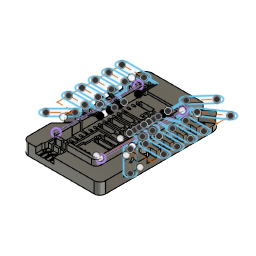
2020_10_06_Nano To Capacitive Sensors One Face Plus v2 (Autodesk Fusion 360 design; units mm, degrees)
Autodesk Fusion 360 part; units mm, degrees
note: some values were not read from the file. Chosen so that the rebuilt part matches the saved one: which face or edge a step refers to. Set by a fixed rule: which sketch regions a step uses.
(part 1 of 3)
sketch "ArduinoNano" plane through (0, 0, 0) normal (0, 0, 1) x (1, 0, 0)
  arc A0 (-13.9477, 42.08) -> (-13.9477, 42.68) centre (-14.2477, 42.38) ccw
  line L0 (-12.5236, 31.2001) -> (-12.133, 30.8096)
  line L1 (-6.271, 43.18) -> (-6.271, 42.88)
  line L2 (-4.5943, 36.68) -> (-4.7943, 36.48)
  line L3 (-13.9477, 42.68) -> (-13.7477, 42.88)
  line L4 (0, 0) -> (0, 43.18)
  line L5 (-6.771, 0) -> (0, 0)
  line L6 (-6.271, 41.88) -> (-6.271, 37.48)
  line L7 (-12.271, 36.18) -> (-12.271, 36.48)
  line L8 (-12.271, 37.48) -> (-12.271, 41.88)
  circle A1 centre (-7.271, 3.0017) radius 0.76
  circle A2 centre (-9.271, 3) radius 0.76
  circle A3 centre (-1.524, 19.156) radius 0.5
  arc A4 (-13.9477, 36.68) -> (-13.9477, 37.28) centre (-14.2477, 36.98) ccw
  line L9 (-6.3515, 30.7521) -> (-5.9609, 31.1427)
  line L10 (-1.524, 24.156) -> (-1.024, 24.156)
  line L11 (-6.271, 36.18) -> (-12.271, 36.18)
  line L12 (-12.271, 36.48) -> (-13.7477, 36.48)
  arc A5 (-13.7477, 37.48) -> (-12.271, 37.48) centre (-13.0093, 38.2183) ccw
  circle A6 centre (-1.524, 11.656) radius 0.5
  arc A7 (-4.7943, 41.88) -> (-6.271, 41.88) centre (-5.5326, 41.1416) ccw
  line L13 (-6.271, 42.88) -> (-4.7943, 42.88)
  line L14 (0, 43.18) -> (-6.271, 43.18)
  circle A8 centre (-1.524, 24.156) radius 0.889
  circle A9 centre (-1.524, 14.156) radius 0.889
  line L15 (-18.542, 43.18) -> (-18.542, 0)
  line L16 (-11.6107, 25.028) -> (-12.0012, 24.6374)
  arc A10 (-13.7477, 42.88) -> (-12.271, 42.88) centre (-13.0093, 43.6183) ccw
  circle A11 centre (-1.524, 9.156) radius 0.5
  circle A12 centre (-17.018, 11.656) radius 0.889
  line L17 (-12.271, 43.18) -> (-18.542, 43.18)
  line L18 (-4.7943, 42.88) -> (-4.5943, 42.68)
  line L19 (-13.7477, 41.88) -> (-13.9477, 42.08)
  arc A13 (-4.7943, 36.48) -> (-6.271, 36.48) centre (-5.5326, 35.7416) ccw
  line L20 (-4.5943, 42.08) -> (-4.7943, 41.88)
  arc A14 (-4.5943, 42.68) -> (-4.5943, 42.08) centre (-4.2943, 42.38) ccw
  line L21 (-6.271, 37.48) -> (-4.7943, 37.48)
  line L22 (-18.542, 0) -> (-11.771, 0)
  arc A15 (-4.5943, 37.28) -> (-4.5943, 36.68) centre (-4.2943, 36.98) ccw
  line L23 (-6.271, 36.48) -> (-6.271, 36.18)
  line L24 (-11.771, 0) -> (-6.771, 0)
  line L25 (-13.7477, 36.48) -> (-13.9477, 36.68)
  line L26 (-13.9477, 37.28) -> (-13.7477, 37.48)
  line L27 (-12.271, 41.88) -> (-13.7477, 41.88)
  line L28 (-4.7943, 37.48) -> (-4.5943, 37.28)
  line L29 (-6.0786, 0) -> (-12.4635, 0)
  circle A16 centre (-7.271, 0.9961) radius 0.76
  arc A17 (-6.8307, 32.2953) -> (-6.8307, 32.0124) centre (-6.9721, 32.1539) cw
  line L30 (-6.771, 13.9686) -> (-11.771, 13.9686)
  line L31 (0, 43.18) -> (-18.542, 43.18)
  line L32 (-12.133, 30.8096) -> (-12.4229, 30.5196)
  line L33 (-18.542, 43.18) -> (0, 43.18)
  circle A18 centre (-17.018, 6.656) radius 0.889
  line L34 (-12.271, 42.88) -> (-12.271, 43.18)
  line L35 (-12.7703, 26.1877) -> (-13.1609, 25.7971)
  line L36 (-6.771, 18.0694) -> (-6.771, 13.9686)
  line L37 (-15.829, 4.2) -> (-2.8014, 4.2)
  circle A19 centre (-1.524, 16.656) radius 0.5
  circle A20 centre (-17.018, 9.156) radius 0.889
  line L38 (-11.9006, 25.3179) -> (-11.6107, 25.028)
  arc A21 (-9.4003, 23.3921) -> (-9.5417, 23.4507) centre (-9.4003, 23.5921) cw
  circle A22 centre (-1.524, 39.156) radius 0.889
  line L39 (-8.0618, 33.5265) -> (-7.9903, 33.4549)
  circle A23 centre (-17.018, 16.656) radius 0.5
  line L40 (-12.4635, 4.2) -> (-6.0786, 4.2)
  circle A24 centre (-17.018, 6.656) radius 0.5
  arc A25 (-14.0589, 28.3093) -> (-14.0003, 28.4507) centre (-13.8589, 28.3093) cw
  line L41 (-5.6781, 31.1427) -> (-5.671, 31.1356)
  circle A26 centre (-17.018, 19.156) radius 0.5
  line L42 (-16.518, 19.156) -> (-17.018, 19.156)
  line L43 (-17.018, 12.156) -> (-17.018, 11.156)
  line L44 (-11.771, 13.9686) -> (-11.771, 18.0694)
  line L45 (-12.4229, 30.5196) -> (-12.8135, 30.9102)
  circle A27 centre (-17.018, 14.156) radius 0.889
  line L46 (-1.524, 19.156) -> (-1.024, 19.156)
  circle A28 centre (-1.524, 9.156) radius 0.889
  line L47 (-12.2912, 24.9274) -> (-11.9006, 25.3179)
  circle A29 centre (-17.018, 31.656) radius 0.889
  circle A30 centre (-1.524, 24.156) radius 0.5
  arc A31 (-12.8065, 31.2001) -> (-12.5236, 31.2001) centre (-12.665, 31.0587) cw
  line L48 (-1.524, 21.656) -> (-1.024, 21.656)
  line L49 (-12.2841, 24.6374) -> (-12.2912, 24.6445)
  arc A32 (-12.2912, 24.6445) -> (-12.2912, 24.9274) centre (-12.1497, 24.7859) cw
  line L50 (-11.771, 18.0694) -> (-6.771, 18.0694)
  circle A33 centre (-17.018, 4.156) radius 0.5
  circle A34 centre (-1.524, 6.656) radius 0.889
  arc A35 (-12.0012, 24.6374) -> (-12.2841, 24.6374) centre (-12.1427, 24.7789) cw
  line L51 (-7.271, 0.2361) -> (-7.271, 1.7561)
  line L52 (-5.671, 30.8528) -> (-6.0616, 30.4622)
  line L53 (-17.518, 11.656) -> (-16.518, 11.656)
  arc A36 (-5.9609, 31.1427) -> (-5.6781, 31.1427) centre (-5.8195, 31.0013) cw
  arc A37 (-12.8135, 30.9102) -> (-12.8135, 31.1931) centre (-12.6721, 31.0517) cw
  line L54 (-12.8135, 31.1931) -> (-12.8065, 31.2001)
  circle A38 centre (-17.018, 16.656) radius 0.889
  arc A39 (-5.671, 31.1356) -> (-5.671, 30.8528) centre (-5.8124, 30.9942) cw
  circle A40 centre (-17.018, 9.156) radius 0.5
  line L55 (-12.4635, 0) -> (-12.4635, 4.2)
  line L56 (-6.0616, 30.4622) -> (-6.3515, 30.7521)
  circle A41 centre (-17.018, 14.156) radius 0.5
  circle A42 centre (-1.524, 16.656) radius 0.889
  line L57 (-7.771, 0.9965) -> (-6.511, 0.9965)
  line L58 (-6.0786, 4.2) -> (-6.0786, 0)
  circle A43 centre (-1.524, 14.156) radius 0.5
  circle A44 centre (-17.018, 11.656) radius 0.5
  arc A45 (-4.5417, 28.4507) -> (-4.4831, 28.3093) centre (-4.6831, 28.3093) cw
  line L59 (-6.8881, 24.0072) -> (-6.8952, 24.0002)
  line L60 (-7.7579, 23.4203) -> (-8.1484, 23.8109)
  arc A46 (-9.0003, 23.4507) -> (-9.1417, 23.3921) centre (-9.1417, 23.5921) cw
  arc A47 (-9.1417, 32.9678) -> (-9.0003, 32.9093) centre (-9.1417, 32.7678) cw
  circle A48 centre (-11.2599, 1.0002) radius 0.76
  line L61 (-12.0199, 1.0002) -> (-10.4999, 1.0002)
  line L62 (-8.3809, 32.7815) -> (-8.7353, 33.1359)
  circle A49 centre (-1.524, 6.656) radius 0.5
  arc A50 (-5.7355, 25.1598) -> (-6.0184, 25.1598) centre (-5.8769, 25.3012) cw
  arc A51 (-7.9903, 33.4549) -> (-7.9903, 33.1721) centre (-8.1317, 33.3135) cw
  line L63 (-9.0003, 32.9093) -> (-4.5417, 28.4507)
  line L64 (-7.2212, 31.6218) -> (-7.5112, 31.9118)
  arc A52 (-6.5407, 31.7225) -> (-6.2579, 31.7225) centre (-6.3993, 31.5811) cw
  line L65 (-7.5112, 31.9118) -> (-7.1206, 32.3023)
  line L66 (-7.2787, 24.6807) -> (-6.8881, 24.2901)
  arc A53 (-13.1609, 25.7971) -> (-13.4437, 25.7971) centre (-13.3023, 25.9385) cw
  arc A54 (-3.9245, 29.3891) -> (-3.9245, 29.1063) centre (-4.0659, 29.2477) cw
  line L67 (-6.5982, 24.58) -> (-6.9888, 24.9706)
  line L68 (-13.4508, 26.087) -> (-13.0602, 26.4776)
  line L69 (-14.0003, 28.4507) -> (-9.5417, 32.9093)
  line L70 (-4.4831, 28.3093) -> (-4.4831, 28.0507)
  line L71 (-6.2579, 31.7225) -> (-6.2508, 31.7154)
  line L72 (-1.524, 34.156) -> (-1.024, 34.156)
  line L73 (-8.7353, 33.1359) -> (-8.3447, 33.5265)
  arc A55 (-7.4105, 32.8751) -> (-7.4105, 32.5923) centre (-7.5519, 32.7337) cw
  line L74 (-9.4003, 32.9678) -> (-9.1417, 32.9678)
  circle A56 centre (-1.524, 31.656) radius 0.5
  circle A57 centre (-1.524, 34.156) radius 0.5
  line L75 (-6.9313, 31.3319) -> (-6.5407, 31.7225)
  line L76 (-13.0602, 26.4776) -> (-12.7703, 26.1877)
  arc A58 (-8.3447, 33.5265) -> (-8.0618, 33.5265) centre (-8.2033, 33.385) cw
  line L77 (-5.4818, 29.8824) -> (-5.7717, 30.1723)
  arc A59 (-7.7004, 32.8822) -> (-7.4176, 32.8822) centre (-7.559, 32.7408) cw
  circle A60 centre (-1.524, 36.656) radius 0.5
  arc A61 (-14.0003, 27.9093) -> (-14.0589, 28.0507) centre (-13.8589, 28.0507) cw
  line L78 (-1.524, 39.156) -> (-1.024, 39.156)
  line L79 (-4.8587, 26.3195) -> (-5.2493, 26.7101)
  line L80 (-6.6414, 31.042) -> (-6.9313, 31.3319)
  arc A62 (-6.2508, 31.7154) -> (-6.2508, 31.4326) centre (-6.3922, 31.574) cw
  line L81 (-4.5417, 27.9093) -> (-9.0003, 23.4507)
  line L82 (-7.4176, 32.8822) -> (-7.4105, 32.8751)
  circle A63 centre (-11.269, 3) radius 0.76
  circle A64 centre (-1.524, 36.656) radius 0.889
  line L83 (-6.2508, 31.4326) -> (-6.6414, 31.042)
  line L84 (-13.4437, 25.7971) -> (-13.4508, 25.8042)
  line L85 (-6.8307, 32.0124) -> (-7.2212, 31.6218)
  arc A65 (-7.1206, 32.3023) -> (-6.8377, 32.3023) centre (-6.9791, 32.1609) cw
  line L86 (-17.518, 6.656) -> (-16.518, 6.656)
  circle A66 centre (-1.524, 4.156) radius 0.889
  line L87 (-7.9903, 33.1721) -> (-8.3809, 32.7815)
  line L88 (-9.1417, 23.3921) -> (-9.4003, 23.3921)
  circle A67 centre (-1.524, 4.156) radius 0.5
  line L89 (-7.4105, 32.5923) -> (-7.8011, 32.2017)
  line L90 (-1.524, 36.656) -> (-1.024, 36.656)
  arc A68 (-13.4508, 25.8042) -> (-13.4508, 26.087) centre (-13.3094, 25.9456) cw
  line L91 (-6.8377, 32.3023) -> (-6.8307, 32.2953)
  line L92 (-9.5417, 23.4507) -> (-14.0003, 27.9093)
  line L93 (-14.0589, 28.0507) -> (-14.0589, 28.3093)
  line L94 (-7.8011, 32.2017) -> (-8.091, 32.4916)
  circle A69 centre (-17.018, 19.156) radius 0.889
  circle A70 centre (-17.018, 34.156) radius 0.889
  arc A71 (-4.4831, 28.0507) -> (-4.5417, 27.9093) centre (-4.6831, 28.0507) cw
  line L95 (-8.091, 32.4916) -> (-7.7004, 32.8822)
  arc A72 (-9.5417, 32.9093) -> (-9.4003, 32.9678) centre (-9.4003, 32.7678) cw
  arc A73 (-4.2214, 29.4032) -> (-3.9386, 29.4032) centre (-4.08, 29.2618) cw
  line L96 (-4.2789, 26.8993) -> (-4.6695, 27.2899)
  arc A74 (-4.5113, 29.976) -> (-4.5113, 29.6931) centre (-4.6528, 29.8345) cw
  arc A75 (-5.1557, 25.7396) -> (-5.4385, 25.7396) centre (-5.2971, 25.8811) cw
  line L97 (-5.7285, 25.1669) -> (-5.7355, 25.1598)
  arc A76 (-4.5759, 26.3195) -> (-4.8587, 26.3195) centre (-4.7173, 26.4609) cw
  arc A77 (-8.0618, 22.8335) -> (-8.3447, 22.8335) centre (-8.2033, 22.9749) cw
  arc A78 (-7.475, 23.4203) -> (-7.7579, 23.4203) centre (-7.6164, 23.5618) cw
  line L98 (-3.9245, 29.1063) -> (-4.3151, 28.7157)
  line L99 (-4.5113, 29.6931) -> (-4.9019, 29.3025)
  line L100 (-6.409, 25.5504) -> (-6.119, 25.8403)
  line L101 (-7.4679, 23.4274) -> (-7.475, 23.4203)
  line L102 (-3.9386, 29.4032) -> (-3.9245, 29.3891)
  line L103 (-5.2493, 26.7101) -> (-4.9594, 27)
  line L104 (-6.6989, 25.2605) -> (-6.3083, 24.8699)
  line L105 (-6.0184, 25.1598) -> (-6.409, 25.5504)
  line L106 (-7.178, 24.0002) -> (-7.5686, 24.3907)
  line L107 (-7.5686, 24.3907) -> (-7.2787, 24.6807)
  line L108 (-4.9594, 27) -> (-4.5688, 26.6094)
  line L109 (-17.018, 37.156) -> (-17.018, 36.156)
  line L110 (-3.9245, 26.9708) -> (-3.996, 26.8993)
  line L111 (-6.9888, 24.9706) -> (-6.6989, 25.2605)
  arc A79 (-6.3154, 24.58) -> (-6.5982, 24.58) centre (-6.4568, 24.7214) cw
  arc A80 (-3.9245, 27.2537) -> (-3.9245, 26.9708) centre (-4.0659, 27.1122) cw
  line L112 (-8.7353, 23.2241) -> (-8.4384, 23.521)
  line L113 (-7.8585, 24.1008) -> (-7.4679, 23.7102)
  line L114 (-5.5392, 26.4201) -> (-5.1486, 26.0296)
  arc A81 (-6.8881, 24.2901) -> (-6.8881, 24.0072) centre (-7.0295, 24.1486) cw
  line L115 (-4.6695, 27.2899) -> (-4.3151, 27.6443)
  line L116 (-4.3151, 27.6443) -> (-3.9245, 27.2537)
  line L117 (-8.0478, 22.8476) -> (-8.0618, 22.8335)
  line L118 (-8.1484, 23.8109) -> (-7.8585, 24.1008)
  arc A82 (-6.8952, 24.0002) -> (-7.178, 24.0002) centre (-7.0366, 24.1416) cw
  arc A83 (-6.3083, 24.8699) -> (-6.3083, 24.5871) centre (-6.4497, 24.7285) cw
  line L119 (-13.3501, 26.7675) -> (-13.7407, 26.3769)
  arc A84 (-7.4679, 23.7102) -> (-7.4679, 23.4274) centre (-7.6094, 23.5688) cw
  arc A85 (-14.3206, 26.9568) -> (-14.6034, 26.9568) centre (-14.462, 27.0982) cw
  arc A86 (-5.3811, 30.5629) -> (-5.0982, 30.5629) centre (-5.2397, 30.4214) cw
  arc A87 (-14.5459, 29.4607) -> (-14.2631, 29.4607) centre (-14.4045, 29.3192) cw
  line L120 (-6.119, 25.8403) -> (-5.7285, 25.4497)
  arc A88 (-8.0478, 23.1304) -> (-8.0478, 22.8476) centre (-8.1892, 22.989) cw
  line L121 (-5.0912, 30.2729) -> (-5.4818, 29.8824)
  line L122 (-6.3083, 24.5871) -> (-6.3154, 24.58)
  arc A89 (-5.0912, 30.5558) -> (-5.0912, 30.2729) centre (-5.2326, 30.4144) cw
  arc A90 (-4.5688, 26.6094) -> (-4.5688, 26.3265) centre (-4.7102, 26.468) cw
  circle A91 centre (-17.018, 24.156) radius 0.5
  circle A92 centre (-17.018, 24.156) radius 0.889
  arc A93 (-11.6539, 32.0699) -> (-11.6539, 32.3527) centre (-11.5125, 32.2113) cw
  line L123 (-5.7717, 30.1723) -> (-5.3811, 30.5629)
  arc A94 (-12.871, 25.2243) -> (-12.871, 25.5072) centre (-12.7296, 25.3658) cw
  arc A95 (-3.996, 26.8993) -> (-4.2789, 26.8993) centre (-4.1375, 27.0407) cw
  line L124 (-4.612, 29.0126) -> (-4.2214, 29.4032)
  line L125 (-4.5688, 26.3265) -> (-4.5759, 26.3195)
  line L126 (-5.0982, 30.5629) -> (-5.0912, 30.5558)
  line L127 (-5.4385, 25.7396) -> (-5.8291, 26.1302)
  arc A96 (-5.7285, 25.4497) -> (-5.7285, 25.1669) centre (-5.8699, 25.3083) cw
  line L128 (-8.4384, 23.521) -> (-8.0478, 23.1304)
  arc A97 (-5.1486, 26.0296) -> (-5.1486, 25.7467) centre (-5.2901, 25.8881) cw
  line L129 (-8.3447, 22.8335) -> (-8.7353, 23.2241)
  line L130 (-5.8291, 26.1302) -> (-5.5392, 26.4201)
  line L131 (-4.3151, 28.7157) -> (-4.612, 29.0126)
  line L132 (-5.1486, 25.7467) -> (-5.1557, 25.7396)
  circle A98 centre (-1.524, 29.156) radius 0.5
  line L133 (-11.5532, 31.3894) -> (-11.8431, 31.0995)
  line L134 (-13.0028, 29.9398) -> (-13.3934, 30.3304)
  arc A99 (-12.2266, 31.78) -> (-11.9438, 31.78) centre (-12.0852, 31.6386) cw
  arc A100 (-11.0741, 32.6497) -> (-11.0741, 32.9326) centre (-10.9326, 32.7911) cw
  line L135 (-13.9732, 30.0334) -> (-13.9661, 30.0405)
  arc A101 (-13.3934, 30.3304) -> (-13.3934, 30.6132) centre (-13.2519, 30.4718) cw
  arc A102 (-14.0306, 26.384) -> (-14.0306, 26.6668) centre (-13.8892, 26.5254) cw
  line L136 (-13.93, 27.3473) -> (-14.3206, 26.9568)
  arc A103 (-13.9732, 29.7506) -> (-13.9732, 30.0334) centre (-13.8318, 29.892) cw
  line L137 (-11.2633, 31.6793) -> (-11.6539, 32.0699)
  line L138 (-14.2269, 28.7157) -> (-14.6175, 29.1063)
  line L139 (-14.0236, 26.3769) -> (-14.0306, 26.384)
  line L140 (-5.1918, 29.5924) -> (-4.8013, 29.983)
  line L141 (-13.3934, 30.6132) -> (-13.3863, 30.6203)
  line L142 (-11.8431, 31.0995) -> (-12.2337, 31.4901)
  line L143 (-1.524, 26.656) -> (-1.024, 26.656)
  line L144 (-11.9438, 31.78) -> (-11.5532, 31.3894)
  arc A104 (-4.8013, 29.983) -> (-4.5184, 29.983) centre (-4.6598, 29.8416) cw
  line L145 (-14.0306, 26.6668) -> (-13.6401, 27.0574)
  line L146 (-13.1034, 30.6203) -> (-12.7129, 30.2297)
  circle A105 centre (-1.524, 26.656) radius 0.889
  arc A106 (-14.6175, 29.1063) -> (-14.6175, 29.3891) centre (-14.4761, 29.2477) cw
  line L147 (-4.5184, 29.983) -> (-4.5113, 29.976)
  line L148 (-11.364, 32.3598) -> (-10.9734, 31.9692)
  line L149 (-14.6034, 26.9568) -> (-14.6175, 26.9708)
  arc A107 (-14.6175, 26.9708) -> (-14.6175, 27.2537) centre (-14.4761, 27.1122) cw
  arc A108 (-12.5811, 25.2173) -> (-12.8639, 25.2173) centre (-12.7225, 25.3587) cw
  arc A109 (-13.7407, 26.3769) -> (-14.0236, 26.3769) centre (-13.8822, 26.5183) cw
  line L150 (-12.2337, 31.7729) -> (-12.2266, 31.78)
  line L151 (-10.9734, 31.9692) -> (-11.2633, 31.6793)
  circle A110 centre (-1.524, 29.156) radius 0.889
  line L152 (-11.6539, 32.3527) -> (-11.6468, 32.3598)
  arc A111 (-11.067, 32.9396) -> (-10.7841, 32.9396) centre (-10.9256, 32.7982) cw
  line L153 (-14.2269, 27.6443) -> (-13.93, 27.3473)
  line L154 (-13.8725, 29.0701) -> (-14.2269, 28.7157)
  line L155 (-14.6175, 29.3891) -> (-14.5459, 29.4607)
  line L156 (-13.6833, 30.0405) -> (-13.2927, 29.6499)
  line L157 (-14.6175, 27.2537) -> (-14.2269, 27.6443)
  line L158 (-12.1905, 25.6079) -> (-12.5811, 25.2173)
  line L159 (-4.9019, 29.3025) -> (-5.1918, 29.5924)
  arc A112 (-13.9661, 30.0405) -> (-13.6833, 30.0405) centre (-13.8247, 29.8991) cw
  line L160 (-12.8639, 25.2173) -> (-12.871, 25.2243)
  line L161 (-12.4804, 25.8978) -> (-12.1905, 25.6079)
  arc A113 (-11.6468, 32.3598) -> (-11.364, 32.3598) centre (-11.5054, 32.2184) cw
  circle A114 centre (-1.524, 26.656) radius 0.5
  arc A115 (-13.3863, 30.6203) -> (-13.1034, 30.6203) centre (-13.2449, 30.4789) cw
  line L162 (-13.2927, 29.6499) -> (-13.5826, 29.36)
  line L163 (-12.7129, 30.2297) -> (-13.0028, 29.9398)
  line L164 (-1.524, 31.656) -> (-1.024, 31.656)
  line L165 (-10.6835, 32.2591) -> (-11.0741, 32.6497)
  line L166 (-10.1611, 23.5785) -> (-9.8067, 23.2241)
  line L167 (-10.4942, 33.5124) -> (-10.4801, 33.5265)
  line L168 (-10.5517, 23.1879) -> (-10.1611, 23.5785)
  line L169 (-10.7841, 32.9396) -> (-10.3935, 32.549)
  circle A116 centre (-1.524, 39.156) radius 0.5
  line L170 (-14.2631, 29.4607) -> (-13.8725, 29.0701)
  circle A117 centre (-17.018, 36.656) radius 0.5
  line L171 (-15.829, 4.2) -> (-15.829, 43.18)
  arc A118 (-10.4801, 33.5265) -> (-10.1973, 33.5265) centre (-10.3387, 33.385) cw
  arc A119 (-12.2337, 31.4901) -> (-12.2337, 31.7729) centre (-12.0923, 31.6315) cw
  circle A120 centre (-17.018, 21.656) radius 0.889
  circle A121 centre (-17.018, 36.656) radius 0.889
  circle A122 centre (-1.524, 11.656) radius 0.889
  circle A123 centre (-17.018, 29.156) radius 0.5
  line L172 (-16.518, 24.156) -> (-17.018, 24.156)
  circle A124 centre (-1.524, 21.656) radius 0.5
  line L173 (-9.8067, 23.2241) -> (-10.1973, 22.8335)
  line L174 (-16.518, 16.656) -> (-17.018, 16.656)
  line L175 (-10.1036, 32.839) -> (-10.4942, 33.2295)
  circle A125 centre (-1.524, 21.656) radius 0.889
  circle A126 centre (-17.018, 29.156) radius 0.889
  line L176 (-17.518, 36.656) -> (-16.518, 36.656)
  line L177 (-13.5826, 29.36) -> (-13.9732, 29.7506)
  line L178 (-1.524, 29.156) -> (-1.024, 29.156)
  line L179 (-10.1973, 33.5265) -> (-9.8067, 33.1359)
  circle A127 centre (-1.524, 34.156) radius 0.9737
  arc A128 (-10.4942, 33.2295) -> (-10.4942, 33.5124) centre (-10.3528, 33.371) cw
  line L180 (-18.542, 0) -> (-18.542, 43.18)
  circle A129 centre (-17.018, 26.656) radius 0.889
  circle A130 centre (-17.018, 26.656) radius 0.5
  line L181 (-11.0308, 24.4482) -> (-11.4214, 24.0576)
  line L182 (-11.7043, 24.0576) -> (-11.7113, 24.0647)
  line L183 (-16.518, 26.656) -> (-17.018, 26.656)
  circle A131 centre (-17.018, 21.656) radius 0.5
  circle A132 centre (-17.018, 31.656) radius 0.5
  line L184 (-11.7113, 24.3475) -> (-11.3207, 24.7381)
  line L185 (-11.1315, 23.7677) -> (-10.7409, 24.1583)
  line L186 (-2.8014, 4.2) -> (-2.8014, 43.18)
  circle A133 centre (-17.018, 39.156) radius 0.889
  circle A134 centre (-1.524, 31.656) radius 0.9737
  circle A135 centre (-1.524, 19.156) radius 0.889
  circle A136 centre (-17.018, 34.156) radius 0.5
  line L187 (-10.7409, 24.1583) -> (-10.451, 23.8684)
  arc A137 (-11.7113, 24.0647) -> (-11.7113, 24.3475) centre (-11.5699, 24.2061) cw
  line L188 (-16.518, 29.156) -> (-17.018, 29.156)
  arc A138 (-11.4214, 24.0576) -> (-11.7043, 24.0576) centre (-11.5628, 24.199) cw
  line L189 (-16.518, 14.156) -> (-17.018, 14.156)
  arc A139 (-10.8416, 23.4778) -> (-11.1244, 23.4778) centre (-10.983, 23.6192) cw
  circle A140 centre (-17.018, 4.156) radius 0.889
  circle A141 centre (-17.018, 39.156) radius 0.5
  line L190 (-13.6401, 27.0574) -> (-13.3501, 26.7675)
  line L191 (-11.0741, 32.9326) -> (-11.067, 32.9396)
  line L192 (-11.3207, 24.7381) -> (-11.0308, 24.4482)
  line L193 (-12.871, 25.5072) -> (-12.4804, 25.8978)
  line L194 (-16.518, 21.656) -> (-17.018, 21.656)
  arc A142 (-10.1973, 22.8335) -> (-10.4801, 22.8335) centre (-10.3387, 22.9749) cw
  line L195 (-10.3935, 32.549) -> (-10.6835, 32.2591)
  line L196 (0, 43.18) -> (0, 0)
  circle A143 centre (-9.271, 0.998) radius 0.76
  arc A144 (-11.1315, 23.4849) -> (-11.1315, 23.7677) centre (-10.9901, 23.6263) cw
  line L197 (-9.8067, 33.1359) -> (-10.1036, 32.839)
  line L198 (-10.4801, 22.8335) -> (-10.5517, 22.905)
  line L199 (-2.024, 11.656) -> (-1.024, 11.656)
  line L200 (-10.451, 23.8684) -> (-10.8416, 23.4778)
  line L201 (-11.1244, 23.4778) -> (-11.1315, 23.4849)
  arc A145 (-10.5517, 22.905) -> (-10.5517, 23.1879) centre (-10.4103, 23.0465) cw
  line L202 (-19.542, 44.18) -> (-19.542, -1)
  line L203 (-19.542, -1) -> (-11.771, -1)
  line L204 (-11.771, -1) -> (-6.771, -1)
  line L205 (-6.771, -1) -> (1, -1)
  line L206 (1, -1) -> (1, 44.18)
  line L207 (1, 44.18) -> (-19.542, 44.18)
  dimension "d482" = 1
sketch "ResistancesHolesTunnels" plane through (0, 0, 0) normal (0, 0, 1) x (1, 0, 0)
  line L0 (-1.524, 39.156) -> (-1.024, 39.156) construction
  line L1 (-1.524, 39.156) -> (-17.018, 39.156) construction
  line L2 (-1.524, 19.156) -> (-17.018, 19.156) construction
  line L3 (-17.018, 21.656) -> (-1.524, 21.656) construction
  line L4 (-1.524, 24.156) -> (-17.018, 24.156) construction
  line L5 (-17.018, 26.656) -> (-1.524, 26.656) construction
  line L6 (-1.524, 29.156) -> (-17.018, 29.156) construction
  line L7 (-17.018, 31.656) -> (-1.524, 31.656) construction
  line L8 (-1.524, 34.156) -> (-1.024, 34.156)
  line L9 (-1.524, 34.156) -> (-10.3687, 34.156) construction
  line L10 (-1.524, 36.656) -> (-10.3687, 36.656) construction
  line L11 (-10.3687, 36.656) -> (-10.3687, 34.156) construction
  line L12 (-17.021, 20.406) -> (-10.021, 20.406)
  line L13 (-10.021, 20.406) -> (-10.021, 17.906)
  line L14 (-10.021, 17.906) -> (-17.021, 17.906)
  line L15 (-17.021, 17.906) -> (-17.021, 20.406)
  line L16 (-17.021, 20.406) -> (-10.021, 17.906) construction
  line L17 (-10.021, 20.406) -> (-17.021, 17.906) construction
  line L18 (-8.521, 22.906) -> (-1.521, 22.906)
  line L19 (-1.521, 22.906) -> (-1.521, 20.406)
  line L20 (-1.521, 20.406) -> (-8.521, 20.406)
  line L21 (-8.521, 20.406) -> (-8.521, 22.906)
  line L22 (-8.521, 22.906) -> (-1.521, 20.406) construction
  line L23 (-1.521, 22.906) -> (-8.521, 20.406) construction
  line L24 (-1.521, 25.406) -> (-8.521, 25.406)
  line L25 (-8.521, 25.406) -> (-8.521, 27.906)
  line L26 (-8.521, 27.906) -> (-1.521, 27.906)
  line L27 (-1.521, 27.906) -> (-1.521, 25.406)
  line L28 (-10.021, 22.906) -> (-17.021, 22.906)
  line L29 (-17.021, 22.906) -> (-17.021, 25.406)
  line L30 (-10.021, 25.406) -> (-10.021, 22.906)
  line L31 (-17.021, 25.406) -> (-10.021, 25.406)
  line L32 (-1.521, 30.406) -> (-8.521, 30.406)
  line L33 (-8.521, 30.406) -> (-8.521, 32.906)
  line L34 (-8.521, 32.906) -> (-1.521, 32.906)
  line L35 (-1.521, 32.906) -> (-1.521, 30.406)
  line L36 (-10.021, 27.906) -> (-17.021, 27.906)
  line L37 (-17.021, 27.906) -> (-17.021, 30.406)
  line L38 (-10.021, 30.406) -> (-10.021, 27.906)
  line L39 (-17.021, 30.406) -> (-10.021, 30.406)
  line L40 (-1.521, 30.406) -> (-8.521, 30.406)
  line L41 (-8.521, 30.406) -> (-8.521, 32.906)
  line L42 (-8.521, 32.906) -> (-1.521, 32.906)
  line L43 (-1.521, 32.906) -> (-1.521, 30.406)
  line L44 (-10.021, 27.906) -> (-17.021, 27.906)
  line L45 (-17.021, 27.906) -> (-17.021, 30.406)
  line L46 (-10.021, 30.406) -> (-10.021, 27.906)
  line L47 (-17.021, 30.406) -> (-10.021, 30.406)
  line L48 (-10.021, 38.006) -> (-17.021, 38.006)
  line L49 (-17.021, 38.006) -> (-17.021, 40.506)
  line L50 (-17.021, 40.506) -> (-10.021, 40.506)
  line L51 (-10.021, 40.506) -> (-10.021, 38.006)
  line L52 (-1.521, 35.506) -> (-8.521, 35.506)
  line L53 (-8.521, 35.506) -> (-8.521, 38.006)
  line L54 (-1.521, 38.006) -> (-1.521, 35.506)
  line L55 (-8.521, 38.006) -> (-1.521, 38.006)
  line L56 (-1.524, 39.556) -> (-17.018, 39.556)
  line L57 (-1.524, 38.756) -> (-17.018, 38.756)
  line L58 (-1.524, 37.056) -> (-10.7687, 37.056)
  line L59 (-10.7687, 37.056) -> (-10.7687, 33.756)
  line L60 (-1.524, 33.756) -> (-10.7687, 33.756)
  line L61 (-1.524, 36.256) -> (-9.9687, 36.256)
  line L62 (-9.9687, 36.256) -> (-9.9687, 34.556)
  line L63 (-1.524, 34.556) -> (-9.9687, 34.556)
  line L64 (-17.018, 31.256) -> (-1.524, 31.256)
  line L65 (-1.524, 29.556) -> (-17.018, 29.556)
  line L66 (-17.018, 26.256) -> (-1.524, 26.256)
  line L67 (-1.524, 24.556) -> (-17.018, 24.556)
  line L68 (-17.018, 21.256) -> (-1.524, 21.256)
  line L69 (-1.524, 19.556) -> (-17.018, 19.556)
  line L70 (-1.524, 18.756) -> (-17.018, 18.756)
  line L71 (-17.018, 22.056) -> (-1.524, 22.056)
  line L72 (-1.524, 23.756) -> (-17.018, 23.756)
  line L73 (-17.018, 27.056) -> (-1.524, 27.056)
  line L74 (-1.524, 28.756) -> (-17.018, 28.756)
  line L75 (-17.018, 32.056) -> (-1.524, 32.056)
  circle A0 centre (-1.524, 39.156) radius 0.4
  circle A1 centre (-17.018, 39.156) radius 0.4
  circle A2 centre (-1.524, 36.656) radius 0.4
  circle A3 centre (-1.524, 34.156) radius 0.4
  circle A4 centre (-1.524, 31.656) radius 0.4
  circle A5 centre (-1.524, 29.156) radius 0.4
  circle A6 centre (-1.524, 26.656) radius 0.4
  circle A7 centre (-1.524, 24.156) radius 0.4
  circle A8 centre (-1.524, 21.656) radius 0.4
  circle A9 centre (-1.524, 19.156) radius 0.4
  circle A10 centre (-17.018, 19.156) radius 0.4
  circle A11 centre (-17.018, 21.656) radius 0.4
  circle A12 centre (-17.018, 24.156) radius 0.4
  circle A13 centre (-17.018, 26.656) radius 0.4
  circle A14 centre (-17.018, 29.156) radius 0.4
  circle A15 centre (-17.018, 31.656) radius 0.4
  line L76 (0, 43.18) -> (-18.542, 43.18)
  line L77 (-18.542, 43.18) -> (-18.542, 0)
  line L78 (-18.542, 0) -> (0, 0)
  line L79 (0, 0) -> (0, 43.18)
  line L80 (-18.542, -2) -> (0, -2)
  line L81 (2, 0) -> (2, 43.18)
  line L82 (0, 45.18) -> (-18.542, 45.18)
  line L83 (-20.542, 43.18) -> (-20.542, 0)
  arc A16 (-18.542, 45.18) -> (-20.542, 43.18) centre (-18.542, 43.18) ccw
  arc A17 (2, 43.18) -> (0, 45.18) centre (0, 43.18) ccw
  arc A18 (0, -2) -> (2, 0) centre (0, 0) ccw
  arc A19 (-20.542, 0) -> (-18.542, -2) centre (-18.542, 0) ccw
  line L84 (0, 43.18) -> (0, 45.18)
  line L85 (-18.542, 43.18) -> (-18.542, 45.18)
  line L86 (0, 45.68) -> (-18.542, 45.68)
  arc A20 (-18.542, 45.68) -> (-21.042, 43.18) centre (-18.542, 43.18) ccw
  line L87 (-21.042, 43.18) -> (-21.042, 0)
  arc A21 (-21.042, 0) -> (-18.542, -2.5) centre (-18.542, 0) ccw
  line L88 (-18.542, -2.5) -> (0, -2.5)
  arc A22 (0, -2.5) -> (2.5, 0) centre (0, 0) ccw
  line L89 (2.5, 0) -> (2.5, 43.18)
  arc A23 (2.5, 43.18) -> (0, 45.68) centre (0, 43.18) ccw
  line L90 (0, 45.18) -> (0, 45.68)
  line L91 (-18.542, 45.18) -> (-18.542, 45.68)
  point P0 (-17.018, 14.156)
  point P1 (-1.524, 19.156)
  point P2 (-17.018, 16.656)
  point P3 (-1.524, 21.656)
  point P4 (-17.018, 19.156)
  point P5 (-1.524, 24.156)
  point P6 (-1.524, 26.656)
  point P7 (-17.018, 21.656)
  point P8 (-1.524, 29.156)
  point P9 (-17.018, 24.156)
  point P10 (-1.524, 31.656)
  point P11 (-17.018, 26.656)
  point P12 (-1.524, 34.156)
  point P13 (-17.018, 29.156)
  point P14 (-1.524, 36.656)
  point P15 (-1.524, 39.156)
  point P16 (-17.018, 31.656)
  point P17 (-17.018, 39.156)
  point P18 (-13.521, 19.156)
  point P19 (-5.021, 21.656)
  point P20 (0, 43.18)
  point P21 (-18.542, 0)
  dimension "d5" = 7
  dimension "d6" = 2.5
  dimension "d7" = 7
  dimension "d8" = 2.5
  dimension "d9" = 7
  dimension "d10" = 2.5
  dimension "d11" = 7
  dimension "d12" = 2.5
  dimension "d13" = 7
  dimension "d14" = 2.5
  dimension "d15" = 7
  dimension "d16" = 2.5
  dimension "d17" = 7
  dimension "d18" = 2.5
  dimension "d19" = 7
  dimension "d20" = 2.5
  dimension "d21" = 7
  dimension "d22" = 2.5
  dimension "d23" = 7
  dimension "d24" = 2.5
  dimension "d27" = 0.4
  dimension "d29" = 0.4
  dimension "d31" = 0.4
  dimension "d32" = 0.4
  dimension "d33" = 0.4
  dimension "d34" = 0.4
  dimension "d35" = 0.4
  dimension "d36" = 0.4
  dimension "d58" = 2
  dimension "d485" = 0.5
  constraint coincident P15 L0.start
  constraint coincident P17 L1.end
  constraint coincident P1 L2.start
  constraint coincident P4 L2.end
  constraint coincident P7 L3.start
  constraint coincident P3 L3.end
  constraint coincident P5 L4.start
  constraint coincident P9 L4.end
  constraint coincident P11 L5.start
  constraint coincident P6 L5.end
  constraint coincident P8 L6.start
  constraint coincident P13 L6.end
  constraint coincident P16 L7.start
  constraint coincident P10 L7.end
  constraint coincident P12 L8.start
  constraint parallel L8 L9
  constraint coincident P14 L10.start
  constraint parallel L9 L10
  constraint perpendicular L9 L11
  constraint horizontal L12
  constraint perpendicular L12 L13
  constraint parallel L12 L14
  constraint parallel L13 L15
  constraint coincident L16 P18
  constraint coincident L17 P18
  constraint horizontal L18
  constraint perpendicular L18 L19
  constraint parallel L18 L20
  constraint parallel L19 L21
  constraint coincident L22 P19
  constraint coincident L23 P19
  constraint horizontal L31
  constraint perpendicular L30 L31
  constraint parallel L28 L31
  constraint parallel L29 L30
  constraint horizontal L26
  constraint perpendicular L26 L27
  constraint parallel L24 L26
  constraint parallel L25 L27
  constraint horizontal L39
  constraint perpendicular L38 L39
  constraint parallel L36 L39
  constraint parallel L37 L38
  constraint horizontal L34
  constraint perpendicular L34 L35
  constraint parallel L32 L34
  constraint parallel L33 L35
  constraint horizontal L47
  constraint perpendicular L46 L47
  constraint parallel L44 L47
  constraint parallel L45 L46
  constraint horizontal L42
  constraint perpendicular L42 L43
  constraint parallel L40 L42
  constraint parallel L41 L43
  constraint horizontal L55
  constraint perpendicular L54 L55
  constraint parallel L52 L55
  constraint parallel L53 L54
  constraint horizontal L50
  constraint perpendicular L50 L51
  constraint parallel L48 L50
  constraint parallel L49 L51
  constraint coincident L56.start A0
  constraint tangent L56 A0
  constraint coincident L56.end A1
  constraint tangent L56 A1
  constraint coincident L58.start A2
  constraint tangent L58 A2
  constraint coincident L63.start A3
  constraint tangent L63 A3
  constraint coincident L75.end A4
  constraint tangent L75 A4
  constraint coincident L65.start A5
  constraint tangent L65 A5
  constraint coincident L73.end A6
  constraint tangent L73 A6
  constraint coincident L67.start A7
  constraint tangent L67 A7
  constraint coincident L71.end A8
  constraint tangent L71 A8
  constraint coincident L69.start A9
  constraint coincident L69.end A10
  constraint tangent L69 A10
  constraint coincident L71.start A11
  constraint tangent L71 A11
  constraint coincident L67.end A12
  constraint tangent L67 A12
  constraint coincident L73.start A13
  constraint tangent L73 A13
  constraint coincident L65.end A14
  constraint tangent L65 A14
  constraint coincident L75.start A15
  constraint tangent L75 A15
  constraint horizontal L76
  constraint vertical L77
  constraint horizontal L78
  constraint vertical L79
  constraint coincident P21 L77.end
  constraint coincident P20 L76.start
  constraint parallel L78 L80
  constraint parallel L79 L81
  constraint parallel L76 L82
  constraint parallel L77 L83
  constraint tangent L83 A16
  constraint tangent L82 A16
  constraint tangent L82 A17
  constraint tangent L81 A17
  constraint equal A16 A17
  constraint tangent L81 A18
  constraint tangent L80 A18
  constraint equal A16 A18
  constraint tangent L80 A19
  constraint tangent L83 A19
  constraint equal A16 A19
  constraint perpendicular L82 L84
  constraint coincident L76.end L77.start
  measures "d5" distance of L13.end L14.end
  measures "d6" distance of L12.end L13.end
  measures "d7" distance of L19.end L20.end
  measures "d8" distance of L18.end L19.end
  measures "d9" distance of L28.start L28.end
  measures "d10" distance of L28.start L30.start
  measures "d11" distance of L24.end L24.start
  measures "d12" distance of L26.end L24.start
  measures "d13" distance of L36.start L36.end
  measures "d14" distance of L38.start L36.start
  measures "d15" distance of L32.start L32.end
  measures "d16" distance of L32.start L34.end
  measures "d17" distance of L36.start L36.end
  measures "d18" distance of L38.start L36.start
  measures "d19" distance of L32.end L32.start
  measures "d20" distance of L34.end L32.start
  measures "d21" distance of L52.start L52.end
  measures "d22" distance of L54.start L52.start
  measures "d23" distance of L48.end L48.start
  measures "d24" distance of L50.end L48.start
  measures "d58" radius of A16
extrude "Extrude1" add sketch "ArduinoNano" along normal blind 9 contours A0 L1 L2 L3 L6 L7 L8 A4 L11 L12 A5 A7 L13 L14 A10 L17 L18 L19 A13 L20 A14 L21 A15 L23 L25 L26 L27 L28 L31 L33 L34 L37 L40 L171 L186 | A0 L1 L2 L3 L6 L7 L8 A4 L11 L12 A5 A7 L13 A10 L18 L19 A13 L20 A14 L21 A15 L23 L25 L26 L27 L28 L31 L33 L34 | L15 L17 L22 L31 L33 L37 L55 L171 L180 | L4 L5 L14 L31 L33 L37 L58 L186 L196 | L5 L22 L24 L29 L37 L40 L55 L58 | L0 L32 L45 A31 A37 L54 | A1 | A2 | A3 | L9 L41 L52 A36 A39 L56 | A6 L199 | A6 L199 | A8 | A9 | L16 L38 L47 L49 A32 A35 | A11 | A12 | A16 L51 L57 | A16 L51 L57 | A16 L51 | A17 L64 L65 L85 A65 L91 | L30 L36 L44 L50 | A18 | L35 A53 L68 L76 L84 A68 | A19 | A20 | A21 A25 A45 A46 A47 L63 L69 L70 L74 A61 L81 L88 L92 L93 A71 A72 | A22 | L39 L62 A51 L73 A58 L87 | A23 | A24 L86 | A24 L86 | A26 | L43 L53 A44 | L43 L53 A44 | L43 L53 A44 | L43 L53 A44 | A27 | A28 | A29 | A30 | A33 | A34 | A38 | A40 | A41 | A42 | A43 | L59 L66 L106 L107 A81 A82 | L60 A78 L101 L113 L118 A84 | A48 L61 | A48 L61 | A49 | A50 L97 L100 L105 L120 A96 | A52 L71 L75 L80 A62 L83 | A54 A73 L98 L102 L124 L131 | L67 L104 L111 A79 A83 L122 | A55 A59 L82 L89 L94 L95 | A56 | A57 | L77 A86 L121 A89 L123 L126 | A60 | L79 A76 L103 L108 A90 L125 | A63 | A64 | A66 | A67 | A69 | A70 | L96 L110 A80 L115 L116 A95 | A74 L99 L140 A104 L147 L159 | A75 L114 L127 A97 L130 L132 | A77 L112 L117 A88 L128 L129 | L109 A117 L176 | L109 A117 L176 | L109 A117 L176 | L109 A117 L176 | L119 A102 L139 L145 A109 L190 | A85 L136 L149 A107 L153 L157 | A87 L138 A106 L154 L155 L170 | A91 | A92 | A93 L137 L148 L151 L152 A113 | A94 A108 L158 L160 L161 L193 | A98 | L133 A99 L142 L144 L150 A119 | L134 A101 L141 L146 A115 L163 | A100 A111 L165 L169 L191 L195 | L135 A103 L156 A112 L162 L177 | A105 | A110 | A114 | L166 L168 L173 A142 L198 A145 | L167 A118 L175 L179 A128 L197 | A116 | A120 | A121 | A122 | A123 | A124 | A125 | A126 | A127 | A129 | A130 | L181 L182 L184 A137 A138 L192 | A131 | A132 | L185 L187 A139 A144 L200 L201 | A133 | A134 | A135 | A136 | A140 | A141 | A143 makes body 1
sketch "Borders" plane through (0, 0, 0) normal (0, 0, 1) x (-1, 0, 0)
  line L0 (28.7609, -40.18) -> (28.7609, 5.8954)
  arc A0 (28.7609, 5.8954) -> (26.7609, 7.8954) centre (26.7609, 5.8954) ccw
  line L1 (26.7609, 7.8954) -> (-7.8139, 7.8954)
  arc A1 (-7.8139, 7.8954) -> (-9.8139, 5.8954) centre (-7.8139, 5.8954) ccw
  line L2 (-9.8139, 5.8954) -> (-9.8139, -40.18)
  line L3 (28.7609, -40.18) -> (28.7609, -51.2538)
  arc A2 (25.7609, -54.2538) -> (28.7609, -51.2538) centre (25.7609, -51.2538) ccw
  line L4 (-9.8139, -40.18) -> (-9.8139, -50.2538)
  line L5 (-5.8139, -54.2538) -> (25.7609, -54.2538)
  arc A3 (-9.8139, -50.2538) -> (-5.8139, -54.2538) centre (-5.8139, -50.2538) ccw
  line L6 (29.7609, -40.18) -> (29.7609, -51.2538)
  arc A4 (25.7609, -55.2538) -> (29.7609, -51.2538) centre (25.7609, -51.2538) ccw
  line L7 (-5.8139, -55.2538) -> (25.7609, -55.2538)
  arc A5 (-10.8139, -50.2538) -> (-5.8139, -55.2538) centre (-5.8139, -50.2538) ccw
  line L8 (-10.8139, -40.18) -> (-10.8139, -50.2538)
  line L9 (-10.8139, 5.8954) -> (-10.8139, -40.18)
  arc A6 (-7.8139, 8.8954) -> (-10.8139, 5.8954) centre (-7.8139, 5.8954) ccw
  line L10 (26.7609, 8.8954) -> (-7.8139, 8.8954)
  arc A7 (29.7609, 5.8954) -> (26.7609, 8.8954) centre (26.7609, 5.8954) ccw
  line L11 (29.7609, -40.18) -> (29.7609, 5.8954)
  dimension "d541" = 4
  dimension "d542" = 1
  constraint tangent L0 A0
  constraint tangent A0 L1
  constraint tangent L1 A1
  constraint tangent A1 L2
  constraint tangent L3 A2
  constraint parallel L2 L4
  constraint tangent A2 L5
  constraint tangent L5 A3
  constraint tangent L4 A3
  measures "d541" radius of A3
extrude "Extrude49" add sketch "Borders" along normal blind 6 contours L0 A0 L1 A1 L2 L3 A2 L4 L5 A3 | L6 A4 L7 A5 L8 L9 A6 L10 A7 L11 bodies 1
extrude "Extrude2" cut sketch "ResistancesHolesTunnels" along normal blind 9 contours L15 A10 | L15 A10 | A9 | L19 A8 | L19 A8 | A11 | L27 A6 | L27 A6 | A13 | L29 A12 | L29 A12 | A7 | L35 L43 A4 | L35 L43 A4 | A15 | L37 L45 A14 | L37 L45 A14 | A5 | L49 A1 | L49 A1 | A0 | L54 A2 | L54 A2 | A3 bodies 1
extrude "Extrude3" add sketch "ResistancesHolesTunnels" against normal blind 6.5 separate body contours L12 L13 L15 L69 A10 | L15 A10 | L15 A10 | L13 L69 L70 A9 | L13 L69 L70 A10 | L13 L14 L15 L70 A10 | A9 | L18 L19 L21 L71 A8 | L21 L68 L71 A8 | L21 L68 L71 A11 | L19 A8 | L19 A8 | L19 L20 L21 L68 A8 | A11 | L24 L25 L27 L66 A6 | L27 A6 | L27 A6 | L25 L66 L73 A13 | L25 L66 L73 A6 | L25 L26 L27 L73 A6 | A13 | L28 L29 L30 L72 A12 | L30 L67 L72 A12 | L30 L67 L72 A7 | L29 A12 | L29 A12 | L29 L30 L31 L67 A12 | A7 | L32 L33 L35 L40 L41 L43 L64 A4 | L35 L43 A4 | L35 L43 A4 | L33 L41 L64 L75 A15 | L33 L41 L64 L75 A4 | L33 L34 L35 L41 L42 L43 L75 A4 | A15 | L36 L37 L38 L44 L45 L46 L74 A14 | L38 L46 L65 L74 A14 | L38 L46 L65 L74 A5 | L37 L45 A14 | L37 L45 A14 | L37 L38 L39 L45 L46 L47 L65 A14 | A5 | L48 L49 L51 L57 A1 | L51 L56 L57 A1 | L51 L56 L57 A0 | L49 A1 | L49 A1 | L49 L50 L51 L56 A1 | A0 | L52 L53 L54 L61 A2 | L54 A2 | L54 A2 | L53 L58 L59 L60 L61 L62 L63 A3 | L53 L58 L61 A2 | L53 L54 L55 L58 A2 | A3 makes body 2 at (-14.1857, 26.256, -2.1667) makes body 3 at (-4.6056, 33.756, -2.1667) makes body 4 at (-14.1857, 31.256, -2.1667) makes body 5 at (-4.3563, 39.556, -4.3333) makes body 6 at (-4.3563, 23.756, -4.3333) makes body 7 at (-4.3563, 18.756, -2.1667) makes body 8 at (-4.3563, 28.756, -4.3333) makes body 9 at (-14.1857, 22.056, -2.1667)
move_body "Move32" bodies 2 7 8 9 3 4 5 6 to x (1, 0, 0) y (0, 1, 0) z (0, 0, 1) at (0, 0, 9)
combine "Combine11" operation cut target body 1 tool bodies 2 7 8 9 3 4 5 6
extrude "Extrude4" add sketch "ResistancesHolesTunnels" along normal blind 9 contours L77 L78 L79 L80 L81 L83 A16 A17 A18 A19 L84 L85 | L76 L82 L84 L85 | L80 L81 L83 A16 A17 A18 A19 A20 L87 A21 L88 A22 L89 A23 L90 L91 | L82 L86 L90 L91 bodies 1
move_body "Move2" bodies 1 to x (1, 0, 0) y (0, 1, 0) z (0, 0, 1) at (0, 0, -9)
extrude "Extrude5" cut sketch "ArduinoNano" against normal blind 4.1 contours L15 L17 L22 L31 L33 L37 L55 L171 L180 | L4 L5 L14 L31 L33 L37 L58 L186 L196 | L5 L22 L24 L29 L37 L40 L55 L58 | A1 | A2 | A3 | A6 L199 | A6 L199 | A8 | A9 | A11 | A12 | A16 L51 L57 | A16 L51 L57 | A16 L51 | A18 | A19 | A20 | A22 | A23 | A24 L86 | A24 L86 | A26 | L43 L53 A44 | L43 L53 A44 | L43 L53 A44 | L43 L53 A44 | A27 | A28 | A29 | A30 | A33 | A34 | A38 | A40 | A41 | A42 | A43 | A48 L61 | A48 L61 | A49 | A56 | A57 | A60 | A63 | A64 | A66 | A67 | A69 | A70 | L109 A117 L176 | L109 A117 L176 | L109 A117 L176 | L109 A117 L176 | A91 | A92 | A98 | A105 | A110 | A114 | A116 | A120 | A121 | A122 | A123 | A124 | A125 | A126 | A127 | A129 | A130 | A131 | A132 | A133 | A134 | A135 | A136 | A140 | A141 | A143 | L202 L203 L204 L205 L206 L207 bodies 1
extrude "Extrude6" cut sketch "ArduinoNano" against normal blind 4.1 contours A0 L1 L2 L3 L6 L7 L8 A4 L11 L12 A5 A7 L13 L14 A10 L17 L18 L19 A13 L20 A14 L21 A15 L23 L25 L26 L27 L28 L31 L33 L34 L37 L40 L171 L186 | A0 L1 L2 L3 L6 L7 L8 A4 L11 L12 A5 A7 L13 A10 L18 L19 A13 L20 A14 L21 A15 L23 L25 L26 L27 L28 L31 L33 L34 | L0 L32 L45 A31 A37 L54 | L9 L41 L52 A36 A39 L56 | L16 L38 L47 L49 A32 A35 | A17 L64 L65 L85 A65 L91 | L30 L36 L44 L50 | L35 A53 L68 L76 L84 A68 | A21 A25 A45 A46 A47 L63 L69 L70 L74 A61 L81 L88 L92 L93 A71 A72 | L39 L62 A51 L73 A58 L87 | L59 L66 L106 L107 A81 A82 | L60 A78 L101 L113 L118 A84 | A50 L97 L100 L105 L120 A96 | A52 L71 L75 L80 A62 L83 | A54 A73 L98 L102 L124 L131 | L67 L104 L111 A79 A83 L122 | A55 A59 L82 L89 L94 L95 | L77 A86 L121 A89 L123 L126 | L79 A76 L103 L108 A90 L125 | L96 L110 A80 L115 L116 A95 | A74 L99 L140 A104 L147 L159 | A75 L114 L127 A97 L130 L132 | A77 L112 L117 A88 L128 L129 | L119 A102 L139 L145 A109 L190 | A85 L136 L149 A107 L153 L157 | A87 L138 A106 L154 L155 L170 | A93 L137 L148 L151 L152 A113 | A94 A108 L158 L160 L161 L193 | L133 A99 L142 L144 L150 A119 | L134 A101 L141 L146 A115 L163 | A100 A111 L165 L169 L191 L195 | L135 A103 L156 A112 L162 L177 | L166 L168 L173 A142 L198 A145 | L167 A118 L175 L179 A128 L197 | L181 L182 L184 A137 A138 L192 | L185 L187 A139 A144 L200 L201 bodies 1
move_body "Move3" bodies 1 to x (1, 0, 0) y (0, 1, 0) z (0, 0, 1) at (0, 0, 9)
move_body "Move28" bodies 1 to x (1, 0, 0) y (0, 1, 0) z (0, 0, 1) at (0, 0, -9)